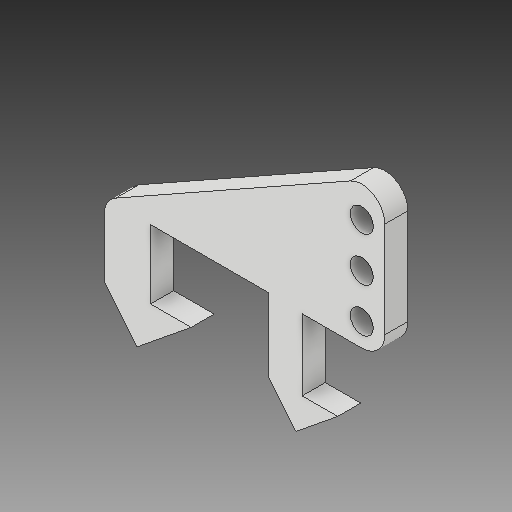
# Autodesk Inventor part: horn
Saved by Autodesk Inventor 2017 (Build 210142000, 142)
## iProperties
Created: 2017-12-26
Part Number: horn
Material: Generic
Document SubType Name: Modeling
Designer: will
Density: 1 g/cm^3
Appearance: Default
Author: will
Autodesk Inventor part; units mm, degrees
ref_plane "YZ Plane" through (0, 0, 0) normal (1, 0, 0) x (0, 1, 0)
ref_plane "XZ Plane" through (0, 0, 0) normal (0, 1, 0) x (-1, 0, 0)
ref_plane "XY Plane" through (0, 0, 0) normal (0, 0, 1) x (1, 0, 0)
sketch "Sketch1" plane through (0, 0, 0) normal (0, 0, 1) x (1, 0, 0)
  line L0 (-89.2878, -36.8646) -> (-89.2878, -45.177)
  line L1 (-112.6031, -46.5773) -> (-92.2694, -35.1221)
  line L2 (-113.6214, -48.3198) -> (-113.6214, -53.3244)
  line L3 (-113.6214, -53.3244) -> (-110.7719, -56.8308)
  line L4 (-110.7719, -56.8308) -> (-106.0759, -53.0146)
  line L5 (-106.0759, -53.0146) -> (-109.5917, -53.0146)
  line L6 (-109.5917, -53.0146) -> (-109.5917, -47.0568)
  line L7 (-96.4553, -47.177) -> (-96.4553, -53.3439)
  line L8 (-96.4553, -53.3439) -> (-93.3742, -53.3439)
  line L9 (-93.3742, -53.3439) -> (-96.9904, -56.2826)
  line L10 (-96.9904, -56.2826) -> (-99.3785, -53.3439)
  line L11 (-99.3785, -53.3439) -> (-99.3785, -47.0568)
  line L12 (-91.2878, -47.177) -> (-96.4553, -47.177)
  line L13 (-99.3785, -47.0568) -> (-109.5917, -47.0568)
  arc A0 (-112.6031, -46.5773) -> (-113.6214, -48.3198) centre (-111.6214, -48.3198) ccw
  arc A1 (-89.2878, -36.8646) -> (-92.2694, -35.1221) centre (-91.2878, -36.8646) ccw
  arc A2 (-91.2878, -47.177) -> (-89.2878, -45.177) centre (-91.2878, -45.177) ccw
  circle A3 centre (-91.2878, -37.5492) radius 1
  circle A4 centre (-91.2878, -41.3631) radius 1
  circle A5 centre (-91.2878, -45.177) radius 1
  line L14 (-91.2878, -45.177) -> (-91.2878, -41.3631) construction
  line L15 (-91.2878, -41.3631) -> (-91.2878, -37.5492) construction
  point P0 (0, 0)
  dimension "d0" = 2
  dimension "d1" = 2
  dimension "d2" = 2
  dimension "d3" = 2
  constraints: 32 end point, 6 centre point, 6 point on circle, 6 tangent, 5 perpendicular, 4 parallel, 3 vertical, 2 collinear, 2 equal radius, 1 coincident, 1 point on line
  measures "d0" radius of A0
  measures "d1" diameter of A3
  measures "d2" diameter of A4
  measures "d3" diameter of A5
extrude "Extrusion1" add sketch "Sketch1" along normal blind 2
body "Solid1"
